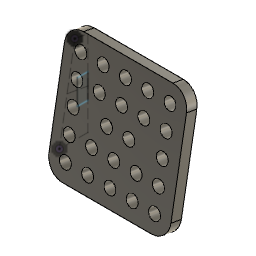
model (Autodesk Fusion 360 design; units mm, degrees)
Autodesk Fusion 360 part; units mm, degrees
sketch "holes" plane through (0, 0, 0) normal (0, 1, 0) x (1, 0, 0) in component "doghome"
  circle A0 centre (28, -28) radius 10
  circle A1 centre (66, -28) radius 10
  circle A2 centre (104, -28) radius 10
  circle A3 centre (142, -28) radius 10
  circle A4 centre (28, -66) radius 10
  circle A5 centre (66, -66) radius 10
  circle A6 centre (104, -66) radius 10
  circle A7 centre (142, -66) radius 10
  circle A8 centre (28, -104) radius 10
  circle A9 centre (66, -104) radius 10
  circle A10 centre (104, -104) radius 10
  circle A11 centre (142, -104) radius 10
  circle A12 centre (28, -142) radius 10
  circle A13 centre (66, -142) radius 10
  circle A14 centre (104, -142) radius 10
  circle A15 centre (142, -142) radius 10
  line L0 (0, 0) -> (208, 0)
  line L1 (208, 0) -> (208, -208)
  line L2 (208, -208) -> (0, -208)
  line L3 (0, -208) -> (0, 0)
  line L4 (28, -28) -> (28, 0) construction
  line L5 (28, -28) -> (0, -28) construction
  circle A16 centre (180, -28) radius 10
  circle A17 centre (180, -66) radius 10
  circle A18 centre (180, -104) radius 10
  circle A19 centre (180, -142) radius 10
  circle A20 centre (28, -180) radius 10
  circle A21 centre (66, -180) radius 10
  circle A22 centre (104, -180) radius 10
  circle A23 centre (142, -180) radius 10
  circle A24 centre (180, -180) radius 10
  arc A25 (0, -180) -> (28, -208) centre (28, -180) ccw
  arc A26 (180, -208) -> (208, -180) centre (180, -180) ccw
  arc A27 (208, -28) -> (180, 0) centre (180, -28) ccw
  arc A28 (28, 0) -> (0, -28) centre (28, -28) ccw
  dimension "d10" = 20
  dimension "d13" = 38
  dimension "d15" = 28
  dimension "d20" = 208
  dimension "d21" = 208
  constraint horizontal L0
  constraint vertical L1
  constraint horizontal L2
  constraint vertical L3
  constraint coincident L0.start L3.end
  constraint coincident A0.centre L4.start
  constraint coincident L0 L4.end
  constraint perpendicular L0 L4
  constraint coincident L3 L5.end
  constraint perpendicular L3 L5
  constraint equal L4 L5
  constraint tangent L2 A25
  constraint coincident L2 A25.end
  constraint coincident L3 A25.start
  constraint tangent L1 A26
  constraint coincident L1 A26.end
  constraint coincident L2 A26.start
  constraint tangent L1 A27
  constraint coincident L1 A27.start
  constraint coincident L0 A27.end
  constraint tangent L0 A28
  constraint tangent L3 A28
  constraint tangent L2 A26
  constraint tangent L3 A25
  constraint tangent L0 A27
  constraint equal A25 A28
  constraint equal A26 A28
  constraint equal A27 A28
  measures "d10" diameter of A0
  measures "d15" distance of A0.centre L4.end
  measures "d20" distance of L0.start L2.end
  measures "d21" distance of L0.start L0.end
sketch "alt holes" plane through (0, 0, 0) normal (0, 1, 0) x (1, 0, 0) in component "doghome"
  circle A0 centre (85, -104) radius 10
  circle A1 centre (123, -104) radius 10
  line L0 (28, -104) -> (85, -104) construction
  line L1 (85, -104) -> (123, -104) construction
  line L2 (123, -104) -> (180, -104) construction
  point P0 (28, -104)
  point P1 (180, -104)
  dimension "d27" = 20
  dimension "d30" = 38
  constraint equal A0 A1
  constraint coincident P0 L0.start
  constraint coincident A0.centre L0.end
  constraint coincident A1.centre L1.end
  constraint horizontal L1
  constraint coincident P1 L2.end
  constraint collinear L0 L1
  constraint equal L0 L2
  measures "d27" diameter of A0
  measures "d30" distance of A0.centre A1.centre
extrude "Extrude1" add sketch "holes" along normal blind 18 contours A9 | A10 | A11 | L0 L1 L2 L3 A25 A26 A27 A28 in component "doghome"
extrude "Extrude2" cut sketch "alt holes" along normal up to surface (18 mm away) in component "doghome"
move_body "Move1" bodies 1 to x (1, 0, 0) y (0, 0.984808, -0.173648) z (0, 0.173648, 0.984808) at (0, 1.0855, 6.1564) in component "doghome"
sketch "Sketch5" plane through (0, 0, 0) normal (1, 0, 0) x (0, 1, 0) in component "doghome"
  line L0 (50.0687, 180.2961) -> (23.6742, 30.6053) construction
  line L1 (50.0687, 180.2961) -> (72.3246, 176.3718) construction
  line L2 (72.3246, 176.3718) -> (72.3246, 30.6053) construction
  line L3 (72.3246, 30.6053) -> (23.6742, 30.6053) construction
  line L4 (36.8715, 105.4507) -> (72.3246, 99.1994) construction
  line L5 (72.3246, 120.3798) -> (54.3246, 120.3798)
  line L6 (54.3246, 120.3798) -> (54.3246, 78.019)
  line L7 (54.3246, 78.019) -> (72.3246, 78.019)
  line L8 (72.3246, 78.019) -> (72.3246, 120.3798)
  point P0 (50.0687, 180.2961)
  point P1 (23.6742, 30.6053)
  dimension "d33" = 36
  dimension "d34" = 18
  constraint coincident P0 L0.start
  constraint coincident P1 L0.end
  constraint perpendicular L0 L1
  constraint vertical L2
  constraint perpendicular L2 L3
  constraint midpoint L0 L4.start
  constraint coincident L2 L4.end
  constraint perpendicular L0 L4
  constraint horizontal L5
  constraint vertical L6
  constraint horizontal L7
  constraint vertical L8
  constraint coincident L2 L5.start
  constraint midpoint L4.end L8
  measures "d33" distance of L4.start L4.end
  measures "d34" distance of L5.start L5.end
component "doghome" placed x (1, 0, 0) y (0, 1, 0) z (0, 0, 1) at (0, 0, 0)
equation "angle = 10 deg"
equation "t = 18 mm"
equation "width = 5"
equation "height = 5"
equation "spacing = 20 mm + t"
equation "d11 = width"
equation "d12 = height"
equation "d13 = spacing"
equation "d14 = -spacing"
equation "d15 = spacing - d10 / 2"
equation "d16 = t"
equation "d20 = 2 * d15 + height * spacing - spacing"
equation "d21 = d15 * 2 + width * spacing - spacing"
equation "d30 = spacing"
equation "d33 = 2 * t"
equation "d34 = t"
